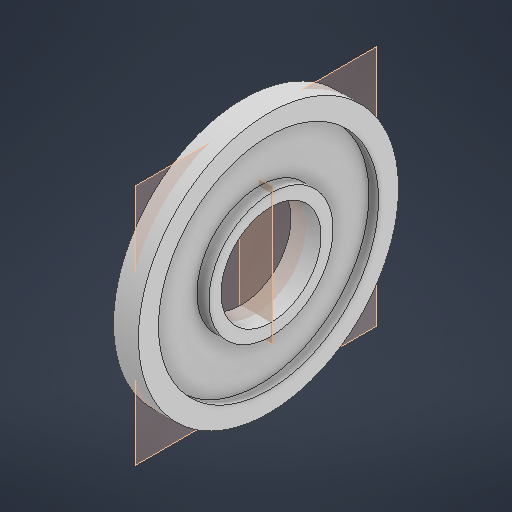
# Autodesk Inventor part: DiscoPaleStadio4-10
Saved by Autodesk Inventor 2026.2 (Build 302298010, 298A)
## iProperties
Created: 2026-04-19
Part Number: DiscoPaleStadio4-10
Material: Generic
Document SubType Name: Modeling
Designer: Yan
Density: 1 g/cm^3
Appearance: Default
Author: Yan
Autodesk Inventor part; units mm, degrees
ref_plane "XZ Plane" through (0, 0, 0) normal (0, 1, 0) x (-1, 0, 0)
sketch "Sketch1" plane through (0, 0, 0) normal (1, 0, 0) x (0, 1, 0)
  circle A0 centre (0, 0) radius 50
  circle A1 centre (0, 0) radius 62
  dimension "d0" = 100
  dimension "d1" = 124
  constraints: 2 centre point, 2 coincident
  measures "d0" diameter of A0
  measures "d1" diameter of A1
extrude "Extrusion1" add sketch "Sketch1" along normal blind 30
ref_plane "Work Plane1" through (0, 0, 0) normal (0, 0, 1) x (1, 0, 0)
sketch "Sketch2" plane through (0, 0, 0) normal (0, 0, 1) x (1, 0, 0)
  line L0 (0, 62) -> (30, 62) projected
  line L1 (18, 62) -> (18, 110)
  line L2 (18, 110) -> (12, 110)
  line L3 (12, 110) -> (12, 62)
  line L4 (0, -62) -> (0, 62) projected
  line L5 (-6, 0) -> (36, 0) projected
  point P0 (0, 0)
  dimension "d5" = 6
  dimension "d6" = 12
  dimension "d7" = 48
  constraints: 6 end point, 3 perpendicular, 2 point on line
  measures "d5" distance between parallel lines of L3 L1
  measures "d6" distance between parallel lines of L4 L3
  measures "d7" distance between parallel lines of L0 L2
revolve "Revolution1" add sketch "Sketch2" angle 360 about axis through (-10, 0, 0) along (1, 0, 0)
ref_plane "Work Plane2" through (15, 0, 0) normal (1, 0, 0) x (0, 1, 0)
sketch "Sketch3" plane through (15, 0, 0) normal (1, 0, 0) x (0, 1, 0)
  circle A0 centre (0, 0) radius 130
  circle A1 centre (0, 0) radius 110
  dimension "d10" = 260
  dimension "d11" = 220
  constraints: 2 centre point, 2 coincident
  measures "d10" diameter of A0
  measures "d11" diameter of A1
extrude "Extrusion2" add sketch "Sketch3" along normal mid plane 25
body "Solid1"
